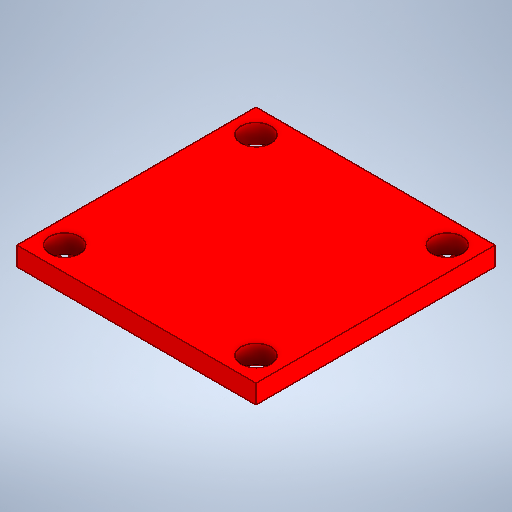
# Autodesk Inventor part: odometry
Saved by Autodesk Inventor 2025 (Build 290162000, 162)
## iProperties
Created: 2025-09-05
Part Number: odometry
Material: 一般
Document SubType Name: Modeling
Designer: sooo1
Density: 1 g/cm^3
Appearance: 既定(1)
Author: sooo1
Autodesk Inventor part; units mm, degrees
ref_plane "YZ Plane" through (0, 0, 0) normal (1, 0, 0) x (0, 1, 0)
ref_plane "XZ Plane" through (0, 0, 0) normal (0, 1, 0) x (-1, 0, 0)
ref_plane "XY Plane" through (0, 0, 0) normal (0, 0, 1) x (1, 0, 0)
sketch "スケッチ1" plane through (0, 0, 0) normal (0, 1, 0) x (-1, 0, 0)
  line L0 (12.7, 12.7) -> (-12.7, 12.7)
  line L1 (-12.7, 12.7) -> (-12.7, -12.7)
  line L2 (-12.7, -12.7) -> (12.7, -12.7)
  line L3 (12.7, -12.7) -> (12.7, 12.7)
  line L4 (12.7, 12.7) -> (-12.7, -12.7) construction
  line L5 (-12.7, 12.7) -> (12.7, -12.7) construction
  circle A0 centre (-10.16, 10.16) radius 1.6
  circle A1 centre (-10.16, -10.16) radius 1.6
  circle A2 centre (10.16, -10.16) radius 1.6
  circle A3 centre (10.16, 10.16) radius 1.6
  point P0 (0, 0)
  dimension "d0" = 25.4
  dimension "d1" = 3.2
  dimension "d2" = 2.54
  dimension "d3" = 2.54
  dimension "d6" = 360
  constraints: 12 end point, 4 centre point, 2 midpoint, 2 parallel, 2 perpendicular, 1 horizontal, 9 other
  measures "d0" distance of L2.end L0.start
  measures "d1" diameter of A0
  measures "d2" distance from line of L1 A0.centre
  measures "d3" distance from line of L0 A0.centre
extrude "押し出し1" add sketch "スケッチ1" along normal blind 2
